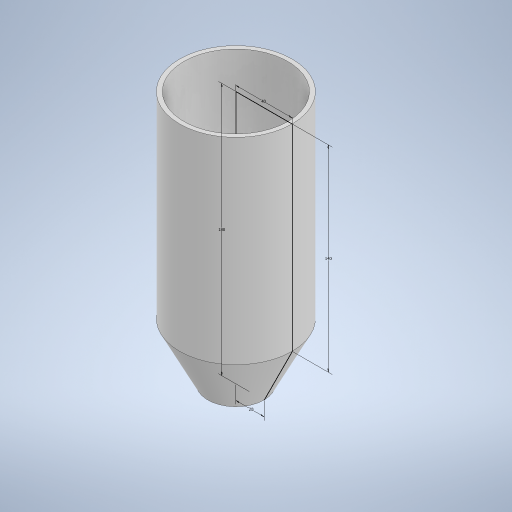
# Autodesk Inventor part: Part2
Saved by Autodesk Inventor 2023.2 (Build 272271030, 271C)
## iProperties
Created: 2024-03-19
Part Number: Part2
Material: Generic
Document SubType Name: Modeling
Designer: ryanv
Density: 1 g/cm^3
Appearance: Default
Author: ryanv
Autodesk Inventor part; units mm, degrees
ref_plane "YZ Plane" through (0, 0, 0) normal (1, 0, 0) x (0, 1, 0)
ref_plane "XZ Plane" through (0, 0, 0) normal (0, 1, 0) x (-1, 0, 0)
ref_plane "XY Plane" through (0, 0, 0) normal (0, 0, 1) x (1, 0, 0)
sketch "Sketch1" plane through (0, 0, 0) normal (0, 0, 1) x (1, 0, 0)
  line L0 (0, 180) -> (40, 180)
  line L1 (40, 180) -> (40, 40)
  line L2 (40, 40) -> (20, 0)
  line L3 (20, 0) -> (0, 0)
  line L4 (0, 0) -> (0, 180)
  point P0 (10, 0)
  dimension "d1" = 40
  dimension "d2" = 20
  dimension "d4" = 180
  dimension "d5" = 140
  constraints: 10 end point, 2 perpendicular, 1 horizontal, 1 midpoint, 1 parallel
  measures "d1" distance between parallel lines of L1 L4
  measures "d2" distance of L2.end L3.end
  measures "d4" distance from line of point (10, 0) L0
  measures "d5" distance from line of L1.end L0
revolve "Revolution1" add sketch "Sketch1" angle 360 about axis through (0, 0, 0) along (0, 1, 0)
sketch "Sketch2" plane through (0, 180, 0) normal (0, 1, 0) x (1, 0, 0)
  circle A0 centre (0, 0) radius 37
  circle A1 centre (0, 0) radius 40 projected
  dimension "d14" = 3
  constraints: 1 centre point, 1 coincident, 1 concentric
  measures "d14" radial gap between concentric circles of A0 A1
extrude "Extrusion1" cut sketch "Sketch2" against normal blind 145 contours A0
sketch "Sketch3" plane through (0, 0, 0) normal (0, -1, 0) x (1, 0, 0)
  circle A0 centre (0, 0) radius 16
  circle A1 centre (0, 0) radius 20 projected
  constraints: 1 centre point, 1 coincident, 1 concentric
extrude "Extrusion2" cut sketch "Sketch3" against normal blind 140 contours A0
sketch "Sketch4" plane through (0, 35, 0) normal (0, 1, 0) x (1, 0, 0)
  circle A0 centre (0, 0) radius 25
  dimension "d11" = 50
  constraints: 1 centre point, 1 coincident
  measures "d11" diameter of A0
extrude "Extrusion3" cut sketch "Sketch4" against normal blind 20
sketch "Sketch5" plane through (0, 0, 0) normal (0, -1, 0) x (1, 0, 0)
  point P0 (0, 0)
body "Solid1"
